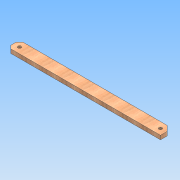
# Autodesk Inventor part: Top_Rear Plank
Saved by Autodesk Inventor 2018.1 (Build 221171000, 171)
## iProperties
Created: 2019-03-15
Part Number: Top_Rear Plank
Material: Wood (Birch)
Document SubType Name: Modeling
Designer: James
Density: 0.55 g/cm^3
Appearance: Birch - Natural Polished
Author: James
Autodesk Inventor part; units mm, degrees
ref_plane "YZ Plane" through (0, 0, 0) normal (1, 0, 0) x (0, 1, 0)
ref_plane "XZ Plane" through (0, 0, 0) normal (0, 1, 0) x (-1, 0, 0)
ref_plane "XY Plane" through (0, 0, 0) normal (0, 0, 1) x (1, 0, 0)
sketch "Sketch1" plane through (0, 0, 0) normal (0, 0, 1) x (1, 0, 0)
  line L0 (0, 0) -> (1930, 0)
  line L1 (1930, 0) -> (1930, 150)
  line L2 (1930, 150) -> (0, 150)
  line L3 (0, 150) -> (0, 0)
  dimension "d0" = 150
  dimension "d1" = 1930
  constraints: 8 end point, 2 parallel, 1 horizontal, 1 perpendicular
  measures "d0" distance of L0.end L1.end
  measures "d1" distance of L1.end L2.end
extrude "Extrusion1" add sketch "Sketch1" along normal blind 50
sketch "Sketch2" plane through (0, 0, 50) normal (0, 0, 1) x (1, 0, 0)
  line L0 (0, 150) -> (0, 0) projected
  line L1 (1930, 0) -> (1930, 150) projected
  point P0 (75, 75)
  point P1 (1855, 75)
  point P2 (0, 75)
  dimension "d4" = 75
  dimension "d5" = 75
  constraints: 2 horizontal alignment, 1 midpoint
  measures "d4" distance from line of point (75, 75) L0
  measures "d5" distance from line of L1 point (1855, 75)
hole "Hole1" at (75, 75, 50) at (1855, 75, 50) direction (0, 0, -1) diameter 30 end through all
chamfer "Chamfer1" distance 5 angle 45 4 edges at (1855, 90, 50) (1855, 90, 0) (75, 90, 50) (75, 90, 0)
chamfer "Chamfer2" distance 65 angle 45 1 edges at (1930, 150, 25) measured on face at (1930, 149.5, 25)
chamfer "Chamfer3" distance 40 angle 45 2 edges at (0, 150, 25) (0, 0, 25)
body "Solid1"
